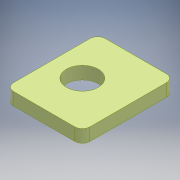
# Autodesk Inventor part: платик под опору редуктора-01
Saved by Autodesk Inventor 2016 (Build 200138000, 138)
## iProperties
Created: 2021-05-08
Part Number: платик под опору редуктора-01
Material: Типовые
Document SubType Name: Modeling
Designer: Лол
Density: 1 g/cm^3
Appearance: Цинк — хромированный 2
Author: Лол
Autodesk Inventor part; units mm, degrees
ref_plane "YZ Plane" through (0, 0, 0) normal (1, 0, 0) x (0, 1, 0)
ref_plane "XZ Plane" through (0, 0, 0) normal (0, 1, 0) x (-1, 0, 0)
ref_plane "XY Plane" through (0, 0, 0) normal (0, 0, 1) x (1, 0, 0)
sketch "Эскиз1" plane through (0, 0, 0) normal (0, 0, 1) x (1, 0, 0)
  line L0 (18, -18) -> (-12, -18)
  line L1 (-12, -18) -> (-12, 18)
  line L2 (-12, 18) -> (18, 18)
  line L3 (18, 18) -> (18, -18)
  circle A0 centre (0, 0) radius 6.25
  dimension "d0" = 36
  dimension "d1" = 12.5
  dimension "d5" = 18
  dimension "d6" = 12
  dimension "d7" = 30
  constraints: 8 end point, 2 parallel, 1 centre point, 1 coincident, 1 horizontal, 1 perpendicular
  measures "d0" distance of L2.end L0.start
  measures "d1" diameter of A0
  measures "d5" distance from line of L2 point (0, 0)
  measures "d6" distance from line of point (0, 0) L1
  measures "d7" distance between parallel lines of L3 L1
extrude "Выдавливание1" add sketch "Эскиз1" along normal blind 5
fillet "Сопряжение1" radius 3 4 edges at (-12, -18, 2.5) (-12, 18, 2.5) (18, 18, 2.5) (18, -18, 2.5)
